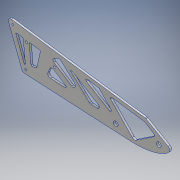
# Autodesk Inventor part: bracket1
Saved by Autodesk Inventor 2018.2 (Build 222227000, 227)
## iProperties
Created: 2018-03-05
Part Number: bracket1
Material: アルミニウム 6061
Document SubType Name: Modeling
Designer: ku_sk
Density: 2.7 g/cm^3
Appearance: アルミニウム - フラット
Mass: 456.161 g
Surface Area: 733.858 cm^2
Volume: 168.949 cm^3
Author: ku_sk
Autodesk Inventor part; units mm, degrees
ref_plane "YZ Plane" through (0, 0, 0) normal (1, 0, 0) x (0, 1, 0)
ref_plane "XZ Plane" through (0, 0, 0) normal (0, 1, 0) x (-1, 0, 0)
ref_plane "XY Plane" through (0, 0, 0) normal (0, 0, 1) x (1, 0, 0)
sketch "スケッチ2" plane through (0, 0, 0) normal (0, 1, 0) x (-1, 0, 0)
  arc A0 (320.7468, 34.8983) -> (392.1215, 71.6787) centre (243.1623, 273.099) ccw projected
  arc A1 (310.5095, 31.8959) -> (320.7468, 34.8983) centre (264.9264, 206.2785) ccw projected
  arc A2 (290.9118, 29.5172) -> (310.5095, 31.8959) centre (291.9468, 102.9093) ccw projected
  arc A3 (278.6891, 31.4878) -> (290.9118, 29.5172) centre (291.5128, 72.1352) ccw projected
  arc A4 (274.9831, 33.389) -> (278.6891, 31.4878) centre (282.4278, 43.3382) ccw projected
  arc A5 (275.4733, 39.2078) -> (274.9831, 33.389) centre (277.0456, 36.1453) ccw projected
  arc A6 (283.1253, 42.3274) -> (275.4733, 39.2078) centre (297.1464, -3.0086) ccw projected
  arc A7 (310.1184, 49.282) -> (283.1253, 42.3274) centre (369.3413, -236.446) ccw projected
  arc A8 (310.1184, 49.282) -> (326.9533, 52.7997) centre (-771.7798, 5269.0252) ccw projected
  arc A9 (326.9533, 52.7997) -> (357.98, 60.8795) centre (256.8539, 385.5961) ccw projected
  arc A10 (357.98, 60.8795) -> (391.1188, 73.3957) centre (268.9975, 346.6028) ccw projected
  arc A11 (392.1215, 71.6787) -> (391.1188, 73.3957) centre (391.5269, 72.4828) ccw projected
  circle A12 centre (287.1934, 37.1564) radius 3 projected
  circle A13 centre (359.7933, 56.2153) radius 3 projected
  arc A14 (100.5026, -29.4375) -> (303.8176, 17.6729) centre (68.6386, 570.3585) ccw projected
  arc A15 (74.9408, -30.0377) -> (100.5026, -29.4375) centre (77.5861, 401.9345) ccw projected
  arc A16 (28.1912, -23.4013) -> (74.9408, -30.0377) centre (76.0159, 145.5175) ccw projected
  arc A17 (1.2395, -11.312) -> (28.1912, -23.4013) centre (55.8939, 74.446) ccw projected
  arc A18 (-6.0217, -4.7376) -> (1.2395, -11.312) centre (16.9451, 13.3315) ccw projected
  arc A19 (-1.6159, 7.4897) -> (-6.0217, -4.7376) centre (0, 0) ccw projected
  arc A20 (17.9572, 9.9554) -> (-1.6159, 7.4897) centre (22.277, -103.2534) ccw projected
  arc A21 (84.7958, 9.311) -> (17.9572, 9.9554) centre (44.6377, -689.2581) ccw projected
  arc A22 (84.7958, 9.311) -> (126.0099, 7.0084) centre (819.0754, 12782.4716) ccw projected
  arc A23 (126.0099, 7.0084) -> (203.0122, 6.466) centre (170.258, 822.6468) ccw projected
  arc A24 (203.0122, 6.466) -> (303.8176, 17.6729) centre (174.1884, 724.7085) ccw projected
  circle A25 centre (20.0666, -1.5588) radius 5 projected
  circle A26 centre (130.4331, -10.1322) radius 5 projected
  line L0 (100.5026, -29.4375) -> (370, -15.1205)
  line L1 (-3.831, 6.6355) -> (54.1787, 40.1274)
  line L2 (1137.2465, 0) -> (-1089.9509, 0) projected
  line L3 (54.1787, 40.1274) -> (410, 89.8795)
  line L4 (370, -15.1205) -> (410, 89.8795)
  point P0 (0, 0)
  point P1 (371.2778, 57.8193)
  dimension "d7" = 30
  dimension "d115" = 370
  dimension "d164" = 40
  dimension "d165" = 105
  constraints: 8 end point, 2 point on circle, 2 tangent
  measures "d7" angle of L2 L1
  measures "d115" horizontal distance of L0.end point (0, 0)
  measures "d164" horizontal distance of L3.end L0.end
  measures "d165" vertical distance of L0.end L3.end
extrude "押し出し3" add sketch "スケッチ2" along normal blind 5 contours A1 A2 A3 A4 A5 A6 A7 A8 A9 A10 A11 A0 | A15 A16 A17 A18 A19 L2 A25 A14 | A14 L2 L4 L0 | L2 A25 A19 A20 A21 A22 A23 A24 A14 | A14 A24 A23 A22 A21 A20 A19 L1 L3 L4 L2
fillet "フィレット2" radius 6 2 edges at (-54.1787, 2.5, 40.1274) (-370, 2.5, -15.1205)
fillet "フィレット2" radius 7 1 edges at (-410, 2.5, 89.8795)
sketch "スケッチ4" plane through (0, 5, 0) normal (0, 1, 0) x (1, 0, 0)
  circle A0 centre (-361.3333, 5.5668) radius 2.5
  line L0 (-53.1667, -39.5431) -> (3.831, -6.6355) projected
  line L1 (-410, -89.8795) -> (-55.3359, -40.2892) projected
  line L2 (-100.5026, 29.4375) -> (-366.1013, 15.3276) projected
  line L3 (-371.3899, 11.472) -> (-410, -89.8795) projected
  circle A1 centre (-394.6339, -77.6337) radius 2.5
  point P0 (0, 0)
  dimension "d21" = 5
  dimension "d22" = 10
  dimension "d23" = 11.5
  dimension "d77" = 10
  dimension "d78" = 10
  dimension "d79" = 5
  constraints: 2 centre point
  measures "d21" diameter of A0
  measures "d22" distance from line of L2 A0.centre
  measures "d23" distance from line of L3 A0.centre
  measures "d77" distance from line of A1.centre L1
  measures "d78" distance from line of L3 A1.centre
  measures "d79" diameter of A1
sketch "スケッチ6" plane through (0, 0, 0) normal (0, -1, 0) x (1, 0, 0)
  circle A0 centre (-20.0666, -1.5588) radius 6
  circle A1 centre (-20.0666, -1.5588) radius 5 projected
  circle A2 centre (-130.4331, -10.1322) radius 6
  circle A3 centre (-130.4331, -10.1322) radius 5 projected
  point P0 (0, 0)
  dimension "d29" = 12
  dimension "d30" = 12
  constraints: 2 centre point, 2 concentric
  measures "d29" diameter of A0
  measures "d30" diameter of A2
extrude "押し出し7" cut sketch "スケッチ6" against normal through all
extrude "押し出し9" cut sketch "スケッチ4" against normal through all
sketch "スケッチ10" plane through (0, 0, 0) normal (0, -1, 0) x (1, 0, 0)
  arc A0 (-243.5017, 17.0901) -> (-236.1351, 26.5049) centre (-240.2302, 22.1197) ccw
  line L0 (-243.5017, 17.0901) -> (-289.7011, 47.1397)
  arc A1 (-289.2417, 55.7878) -> (-289.7011, 47.1397) centre (-286.9749, 51.3311) ccw
  line L1 (-289.2417, 55.7878) -> (-278.2813, 61.3624)
  arc A2 (-272.602, 60.56) -> (-278.2813, 61.3624) centre (-276.0146, 56.9057) ccw
  line L2 (-272.602, 60.56) -> (-236.1351, 26.5049)
  arc A3 (-197.7105, 2.9358) -> (-194.5631, 1.5972) centre (-194.2979, 6.5902) ccw
  line L3 (-197.7105, 2.9358) -> (-245.7449, 47.7935)
  arc A4 (-243.3486, 50.9688) -> (-245.7449, 47.7935) centre (-244.3799, 49.2552) ccw
  line L4 (-243.3486, 50.9688) -> (-175.2771, 10.0005)
  arc A5 (-178.1207, 0.7236) -> (-175.2771, 10.0005) centre (-177.8554, 5.7166) ccw
  line L5 (-178.1207, 0.7236) -> (-194.5631, 1.5972)
  arc A6 (-261.0576, 5.1301) -> (-259.2627, 10.6407) centre (-260.8985, 8.1258) ccw
  line L6 (-261.0576, 5.1301) -> (-298.4553, 7.117)
  arc A7 (-304.5255, 16.8469) -> (-298.4553, 7.117) centre (-298.0839, 14.1072) ccw
  line L7 (-304.5255, 16.8469) -> (-300.05, 27.3695)
  arc A8 (-289.7917, 30.4977) -> (-300.05, 27.3695) centre (-293.6084, 24.6298) ccw
  line L8 (-289.7917, 30.4977) -> (-259.2627, 10.6407)
  arc A9 (-365.392, 5.0895) -> (-362.4981, 5.7767) centre (-363.9903, 5.6235) ccw
  line L9 (-365.392, 5.0895) -> (-386.8582, 61.4391)
  arc A10 (-384.7123, 64.1318) -> (-386.8582, 61.4391) centre (-384.9892, 62.1511) ccw
  line L10 (-384.7123, 64.1318) -> (-369.8076, 62.0477)
  arc A11 (-368.095, 60.2713) -> (-369.8076, 62.0477) centre (-370.0845, 60.067) ccw
  line L11 (-368.095, 60.2713) -> (-362.4981, 5.7767)
  arc A12 (-203.9352, 51.8756) -> (-205.8976, 46.3341) centre (-204.3507, 48.9045) ccw
  line L12 (-203.9352, 51.8756) -> (-174.9447, 47.8219)
  arc A13 (-173.2007, 46.9332) -> (-174.9447, 47.8219) centre (-175.3602, 44.8508) ccw
  line L13 (-173.2007, 46.9332) -> (-142.4229, 15.0159)
  arc A14 (-146.1294, 10.363) -> (-142.4229, 15.0159) centre (-144.5824, 12.9334) ccw
  line L14 (-146.1294, 10.363) -> (-205.8976, 46.3341)
  arc A15 (-350.4293, 59.3381) -> (-352.6958, 57.153) centre (-350.7063, 57.3574) ccw
  line L15 (-350.4293, 59.3381) -> (-325.6702, 55.876)
  arc A16 (-323.9981, 53.4468) -> (-325.6702, 55.876) centre (-325.9472, 53.8953) ccw
  line L16 (-323.9981, 53.4468) -> (-332.6963, 15.6506)
  arc A17 (-336.2021, 11.9623) -> (-332.6963, 15.6506) centre (-337.5689, 16.7719) ccw
  line L17 (-336.2021, 11.9623) -> (-345.4257, 9.3412)
  arc A18 (-347.9619, 11.0607) -> (-345.4257, 9.3412) centre (-345.9724, 11.265) ccw
  line L18 (-347.9619, 11.0607) -> (-352.6958, 57.153)
  arc A19 (-141.2249, 43.1068) -> (-143.7999, 38.0533) centre (-141.6404, 40.1357) ccw
  line L19 (-141.2249, 43.1068) -> (-57.0439, 31.3359)
  arc A20 (-55.8272, 30.882) -> (-57.0439, 31.3359) centre (-57.4593, 28.3648) ccw
  line L20 (-55.8272, 30.882) -> (-31.9951, 15.4288)
  arc A21 (-31.9514, 10.4234) -> (-31.9951, 15.4288) centre (-33.6272, 12.9117) ccw
  line L21 (-31.9514, 10.4234) -> (-78.0412, -20.6163)
  arc A22 (-88.2687, -19.5339) -> (-78.0412, -20.6163) centre (-82.51, -13.9808) ccw
  line L22 (-88.2687, -19.5339) -> (-143.7999, 38.0533)
  circle A23 centre (-361.3333, -5.5648) radius 2.5
  circle A24 centre (-394.6334, 77.6359) radius 2.5
  arc A25 (-398.2739, 88.2422) -> (-405.7847, 78.8177) centre (-399.2433, 81.3096) ccw
  line L23 (-371.3899, -11.47) -> (-405.7847, 78.8177)
  arc A26 (-371.3899, -11.47) -> (-366.1013, -15.3256) centre (-365.783, -9.3341) ccw
  line L24 (-100.5028, -29.4369) -> (-366.1013, -15.3256)
  arc A27 (-100.5028, -29.4369) -> (-74.941, -30.0373) centre (-77.5839, 401.9349) ccw
  arc A28 (-74.941, -30.0373) -> (-28.1913, -23.4012) centre (-76.0151, 145.5179) ccw
  arc A29 (-28.1913, -23.4012) -> (-1.2396, -11.312) centre (-55.8935, 74.4463) ccw
  arc A30 (-1.2396, -11.312) -> (6.0217, -4.7376) centre (-16.945, 13.3316) ccw
  arc A31 (6.0217, -4.7376) -> (3.831, 6.6355) centre (0, 0) ccw
  line L25 (-53.1665, 39.5434) -> (3.831, 6.6355)
  arc A32 (-53.1665, 39.5434) -> (-55.3356, 40.2895) centre (-56.1665, 34.3473) ccw
  line L26 (-398.2739, 88.2422) -> (-55.3356, 40.2895)
  circle A33 centre (-287.1932, 37.158) radius 3
  circle A34 centre (-359.793, 56.2173) radius 3
  point P0 (0, 0)
  constraints: 62 point on circle, 54 end point, 35 centre point
extrude "押し出し13" cut sketch "スケッチ10" against normal through all contours L0 A1 L1 A2 L2 A0 | L3 A4 L4 A5 L5 A3 | L6 A7 L7 A8 L8 A6 | L9 A10 L10 A11 L11 A9 | L12 A13 L13 A14 L14 A12 | L15 A16 L16 A17 L17 A18 L18 A15 | L19 A20 L20 A21 L21 A22 L22 A19
